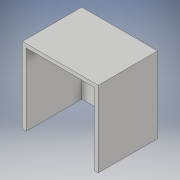
# Autodesk Inventor part: Gehäuse Motor
Saved by Autodesk Inventor 2018 (Build 220112000, 112)
## iProperties
Created: 2018-01-20
Part Number: Gehäuse Motor
Material: Generisch
Document SubType Name: Blech
Designer: Andreas
Density: 1 g/cm^3
Sheet Metal Rule: Standard_mm
Appearance: Vorgabe
Author: Andreas
Autodesk Inventor part; units mm, degrees
ref_plane "YZ Plane" through (0, 0, 0) normal (1, 0, 0) x (0, 1, 0)
ref_plane "XZ Plane" through (0, 0, 0) normal (0, 1, 0) x (-1, 0, 0)
ref_plane "XY Plane" through (0, 0, 0) normal (0, 0, 1) x (1, 0, 0)
sketch "Skizze1" plane through (0, 0, 0) normal (0, 1, 0) x (-1, 0, 0)
  line L0 (0, 0) -> (30, 0)
  line L1 (30, 0) -> (30, 30)
  line L2 (30, 30) -> (0, 30)
  line L3 (0, 30) -> (0, 0)
  circle A0 centre (15, 15) radius 14.1
  dimension "d7" = 28.2
  dimension "d20" = 30
  dimension "d21" = 30
  constraints: 8 end point, 2 parallel, 1 centre point, 1 horizontal, 1 perpendicular
  measures "d7" diameter of A0
  measures "d20" distance of L2.end L0.start
  measures "d21" distance of L1.end L2.end
extrude "Extrusion1" add sketch "Skizze1" along normal blind 22 contours L3 L2 L1 L0 | A0
sketch "Skizze2" plane through (0, 22, 0) normal (0, 1, 0) x (1, 0, 0)
  line L0 (0, 0) -> (-30, 0) projected
  line L1 (-1.5, 0) -> (-28.5, 0)
  line L2 (-28.5, 0) -> (-28.5, -28.5)
  line L3 (-28.5, -28.5) -> (-1.5, -28.5)
  line L4 (-1.5, -28.5) -> (-1.5, 0)
  line L5 (-30, 0) -> (-30, -30) projected
  line L6 (0, -30) -> (0, 0) projected
  line L7 (-30, -30) -> (0, -30) projected
  dimension "d8" = 1.5
  dimension "d9" = 1.5
  dimension "d10" = 1.5
  constraints: 8 end point, 2 parallel, 1 horizontal, 1 perpendicular, 1 point on line
  measures "d8" distance between parallel lines of L5 L2
  measures "d9" distance between parallel lines of L6 L4
  measures "d10" distance between parallel lines of L3 L7
extrude "Extrusion2" cut sketch "Skizze2" against normal blind 22 contours L4 L3 L2 L0
sketch "Skizze5" plane through (0, 22, 0) normal (0, 1, 0) x (1, 0, 0)
  line L0 (-30, 0) -> (-30, -30) projected
  line L1 (0, 0) -> (-30, 0)
  line L2 (-30, 0) -> (-30, -30)
  line L3 (-30, -30) -> (0, -30)
  line L4 (0, -30) -> (0, 0)
  line L5 (-31.5556, 0) -> (-1.5, 0) construction
  circle A0 centre (-15, -15) radius 1.35
  line L6 (-1.5, -28.5) -> (-28.5, -28.5) projected
  line L7 (-1.5, 0) -> (-1.5, -28.5)
  line L8 (-28.5, -28.5) -> (-28.5, 0) projected
  line L9 (-1.5, -28.5) -> (-28.5, -28.5)
  dimension "d17" = 2.7
  constraints: 14 end point, 2 parallel, 2 perpendicular, 1 centre point, 1 horizontal, 1 point on line, 1 vertical
  measures "d17" diameter of A0
extrude "Extrusion4" add sketch "Skizze5" along normal blind 1.5
equation "\"Biegeradius\" = Stärke"
equation "\"BreiteBiegungsfreistellung\" = Stärke"
equation "\"TiefeBiegungsfreistellung\" = 0.5 * Stärke"
equation "\"GrößeEckenfreistellung\" = 4 * Stärke"
equation "\"MinimalRest\" = 2 * Stärke"
equation "\"Übergangsradius\" = Biegeradius"
equation "\"JacobiRadiusGröße\" = Biegeradius"
equation "\"Abstandsgröße\" = Stärke"
equation "\"Stärke\" = 0.5"
